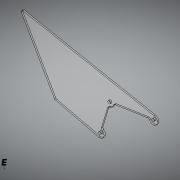
# Autodesk Inventor part: 前足カバー
Saved by Autodesk Inventor 2019 (Build 230136000, 136)
## iProperties
Created: 2019-09-18
Part Number: 前足カバー
Material: ポリカーボネート、クリア
Document SubType Name: Modeling
Designer: tanjihayato
Density: 1.2 g/cm^3
Appearance: ポリカーボネート - クリア
Author: tanjihayato
Autodesk Inventor part; units mm, degrees
ref_plane "YZ Plane" through (0, 0, 0) normal (1, 0, 0) x (0, 1, 0)
ref_plane "XZ Plane" through (0, 0, 0) normal (0, 1, 0) x (-1, 0, 0)
ref_plane "XY Plane" through (0, 0, 0) normal (0, 0, 1) x (1, 0, 0)
sketch "スケッチ1" plane through (0, 0, 0) normal (0, 0, 1) x (1, 0, 0)
  circle A0 centre (70.4743, -10.4118) radius 1.5
  circle A1 centre (127.6431, 30.2622) radius 1.5
  circle A2 centre (80.4743, 23.124) radius 1.5
  arc A3 (123.1938, 29.5888) -> (128.4956, 34.6807) centre (127.6431, 30.2622) ccw
  arc A4 (79.1884, 18.8116) -> (84.9237, 23.7973) centre (80.4743, 23.124) ccw
  arc A5 (69.4242, -14.7876) -> (71.7602, -6.0994) centre (70.4743, -10.4118) ccw
  line L0 (79.1884, 18.8116) -> (71.7602, -6.0994)
  line L1 (84.9237, 23.7973) -> (123.1938, 29.5888)
  circle A6 centre (-12.3701, 60.3295) radius 1.5
  line L2 (-12.086, 61.8023) -> (128.4956, 34.6807)
  line L3 (-13.6756, 59.5908) -> (21.6449, -2.8307)
  circle A7 centre (22.9504, -2.092) radius 1.5
  line L4 (22.6004, -3.5506) -> (69.4242, -14.7876)
  line L5 (69.4242, -14.7876) -> (108.6075, -24.1909)
  point P0 (0, 0)
  point P1 (0, 0)
  dimension "d0" = 3
  dimension "d1" = 3
  dimension "d2" = 4.5
  dimension "d3" = 4.5
  constraints: 13 end point, 10 point on circle, 8 centre point, 6 tangent, 4 point on line, 3 coincident, 1 collinear, 4 other
  measures "d0" diameter of A6
  measures "d1" diameter of A7
  measures "d2" radius of A4
  measures "d3" radius of A3
extrude "押し出し1" add sketch "スケッチ1" along normal blind 1.5
fillet "フィレット1" radius 2 4 edges at (84.9237, 23.7973, 0.75) (79.1884, 18.8116, 0.75) (71.7602, -6.0994, 0.75) (123.1938, 29.5888, 0.75)
